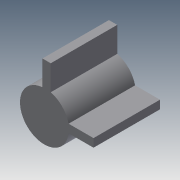
# Autodesk Inventor part: work planes
Saved by Autodesk Inventor 2013 (Build 170138000, 138)
## iProperties
Created: 2013-11-12
Part Number: work planes
Material: Generic
Document SubType Name: Modeling
Designer: Thendric
Density: 1 g/cm^3
Author: Thendric
Autodesk Inventor part; units mm, degrees
ref_plane "YZ Plane" through (0, 0, 0) normal (1, 0, 0) x (0, 1, 0)
ref_plane "XZ Plane" through (0, 0, 0) normal (0, 1, 0) x (-1, 0, 0)
ref_plane "XY Plane" through (0, 0, 0) normal (0, 0, 1) x (1, 0, 0)
sketch "Sketch1" plane through (0, 0, 0) normal (0, 0, 1) x (1, 0, 0)
  line L0 (3.1527, 12.1031) -> (3.1527, 31.2795)
  line L1 (3.1527, 31.2795) -> (-3.1973, 31.2795)
  line L2 (-3.1973, 31.2795) -> (-3.1973, 12.2295)
  line L3 (16.78, -1.8883) -> (35.83, -1.8883)
  line L4 (35.83, -1.8883) -> (35.83, -8.2383)
  line L5 (35.83, -8.2383) -> (16.7392, -8.2383)
  arc A0 (16.78, -1.8883) -> (3.1527, 12.1031) centre (-1.7509, -6.305) ccw
  arc A1 (-3.1973, 12.2295) -> (16.7392, -8.2383) centre (-1.7509, -6.305) ccw
  point P0 (0, 0)
  dimension "d0" = 19.05
  dimension "d2" = 19.05
  dimension "d3" = 19.05
  dimension "d4" = 6.35
  dimension "d5" = 6.35
  constraints: 12 end point, 4 point on circle, 2 centre point, 2 parallel, 1 horizontal, 1 perpendicular
  measures "d0" distance of L1.end L2.end
  measures "d2" radius of A0
  measures "d3" distance of L3.end L3.start
  measures "d4" distance of L1.end L0.end
  measures "d5" distance of L4.end L3.end
extrude "Extrusion1" add sketch "Sketch1" along normal blind 50.8
body "Solid1"
